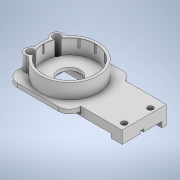
# Autodesk Inventor part: мотор_плеча_1.1
Saved by Autodesk Inventor 2022 (Build 260153000, 153)
## iProperties
Created: 2022-12-03
Part Number: мотор_плеча_1.1
Material: Типовые
Document SubType Name: Modeling
Designer: Папа
Density: 1 g/cm^3
Appearance: По умолчанию
Author: Папа
Autodesk Inventor part; units mm, degrees
ref_plane "YZ Plane" through (0, 0, 0) normal (1, 0, 0) x (0, 1, 0)
ref_plane "XZ Plane" through (0, 0, 0) normal (0, 1, 0) x (-1, 0, 0)
ref_plane "XY Plane" through (0, 0, 0) normal (0, 0, 1) x (1, 0, 0)
sketch "Эскиз1" plane through (0, 0, 0) normal (0, 1, 0) x (-1, 0, 0)
  arc A0 (-2.6622, -14.05) -> (-2.6622, 14.05) centre (0, 0) ccw
  line L0 (-2.6622, 14.05) -> (-34.2422, 14.05)
  line L1 (-34.2422, -14.05) -> (-2.6622, -14.05)
  arc A1 (-34.2422, 6.025) -> (-34.2422, -6.025) centre (-34.2422, 0) ccw
  line L2 (0, 0) -> (-101.5894, 0) construction
  line L3 (-34.2422, 14.05) -> (-34.2422, 6.025)
  line L4 (-34.2422, -6.025) -> (-34.2422, -14.05)
  line L5 (-52.75, 14.55) -> (22.25, 14.55)
  line L6 (22.25, 14.55) -> (22.25, -14.55)
  line L7 (22.25, -14.55) -> (-52.75, -14.55)
  line L8 (-52.75, -14.55) -> (-52.75, 14.55)
  line L9 (-52.75, 14.55) -> (22.25, -14.55) construction
  line L10 (22.25, 14.55) -> (-52.75, -14.55) construction
  line L11 (14.3, 0) -> (22.25, 0)
  line L12 (-34.2422, 6.025) -> (-34.2422, -6.025) construction
  line L13 (22.25, -14.55) -> (-52.75, -14.55)
  line L14 (-52.75, -14.55) -> (-52.75, -17.55)
  line L15 (-52.75, -17.55) -> (22.25, -17.55)
  line L16 (22.25, -17.55) -> (22.25, -14.55)
  point P0 (-15.25, 0)
  dimension "d0" = 28.6
  dimension "d2" = 12.05
  dimension "d4" = 31.58
  dimension "d5" = 14.05
  dimension "d9" = 29.1
  dimension "d10" = 75
  dimension "d12" = 3
  dimension "d25" = 22.25
  constraints: 34 end point, 5 horizontal, 5 point on circle, 4 collinear, 4 midpoint, 4 parallel, 4 perpendicular, 2 centre point, 2 point on line, 1 coincident
  measures "d0" diameter of A0
  measures "d2" diameter of A1
  measures "d4" distance of L1.start L1.end
  measures "d5" distance between parallel lines of L1 L2
  measures "d9" distance between parallel lines of L5 L7
  measures "d10" distance of L6.end L7.end
  measures "d12" distance of L15.end L6.end
  measures "d25" distance from line of L6 point (0, 0)
extrude "Выдавливание2" add sketch "Эскиз1" along normal blind 4
sketch "Эскиз2" plane through (0, 4, 0) normal (0, 1, 0) x (1, 0, 0)
  circle A0 centre (-18.75, -9.5) radius 2.05
  circle A1 centre (-18.75, 9.5) radius 2.05
  circle A2 centre (49.25, -9.5) radius 2.05
  circle A3 centre (49.25, 9.5) radius 2.05
  line L0 (-18.75, -9.5) -> (49.25, -9.5) construction
  line L1 (49.25, -9.5) -> (49.25, 9.5) construction
  line L2 (49.25, 9.5) -> (-18.75, 9.5) construction
  line L3 (-18.75, 9.5) -> (-18.75, -9.5) construction
  line L4 (52.75, -14.55) -> (52.75, 17.55) projected
  line L5 (52.75, -14.55) -> (52.75, 17.55)
  line L6 (-22.25, 17.55) -> (-22.25, -14.55) projected
  line L7 (-22.25, -14.55) -> (52.75, -14.55) projected
  line L8 (34.2422, -14.05) -> (2.6622, -14.05) projected
  line L9 (2.6622, 14.05) -> (34.2422, 14.05) projected
  line L10 (2.6622, -14.05) -> (2.6622, 14.05) construction
  line L11 (2.6622, 0) -> (-18.75, 0)
  point P0 (0, 0)
  dimension "d15" = 4.1
  dimension "d16" = 19
  dimension "d17" = 68
  dimension "d21" = 3.5
  constraints: 14 end point, 4 centre point, 3 equal radius, 2 coincident, 2 midpoint, 2 parallel, 2 perpendicular, 1 horizontal, 1 vertical
  measures "d15" diameter of A0
  measures "d16" distance of L2.end L0.start
  measures "d17" distance of L1.end L2.end
  measures "d21" distance between parallel lines of L6 L3
extrude "Выдавливание3" cut sketch "Эскиз2" against normal blind 4.1
sketch "Эскиз9" plane through (0, 4, 0) normal (0, 1, 0) x (1, 0, 0)
  circle A0 centre (-18.75, -9.5) radius 2.05 projected
  circle A1 centre (-18.75, -9.5) radius 2.05
  circle A2 centre (-18.75, 9.5) radius 2.05 projected
  circle A3 centre (-18.75, 9.5) radius 2.05
  circle A4 centre (49.25, 9.5) radius 2.05 projected
  circle A5 centre (49.25, 9.5) radius 2.05
  circle A6 centre (49.25, -9.5) radius 2.05 projected
  circle A7 centre (49.25, -9.5) radius 2.05
  line L0 (-22.25, -14.55) -> (52.75, -14.55) projected
  line L1 (52.75, -14.55) -> (52.75, 17.55) projected
  line L2 (-22.25, -14.55) -> (52.75, -14.55)
  line L3 (52.75, -14.55) -> (52.75, 17.55)
  line L4 (52.75, 17.55) -> (-22.25, 17.55)
  line L5 (-22.25, 17.55) -> (-22.25, -14.55)
  circle A8 centre (0, 0) radius 8
  line L6 (-18.75, -9.5) -> (-18.75, 9.5) construction
  line L7 (34.2422, -14.05) -> (2.6622, -14.05) projected
  line L8 (2.6622, 14.05) -> (34.2422, 14.05) projected
  line L9 (10.1489, -14.05) -> (10.1489, 14.05)
  dimension "d70" = 16
  dimension "d120" = 18.75
  constraints: 12 end point, 5 centre point, 4 coincident, 2 parallel, 2 perpendicular, 2 point on line, 1 horizontal, 1 vertical
  measures "d70" diameter of A8
  measures "d120" distance from line of A8.centre L6
extrude "Выдавливание11" add sketch "Эскиз9" along normal blind 2.1
sketch "Эскиз10" plane through (0, 0, 0) normal (0, -1, 0) x (1, 0, 0)
  line L0 (52.75, -17.55) -> (-22.25, -17.55) projected
  line L1 (-22.25, -17.55) -> (52.75, -17.55)
  line L2 (52.75, -17.55) -> (52.75, 14.55)
  line L3 (52.75, 14.55) -> (-22.25, 14.55)
  line L4 (-22.25, 14.55) -> (-22.25, -17.55)
  circle A0 centre (-18.75, -9.5) radius 2.05 projected
  circle A1 centre (-18.75, -9.5) radius 2.05
  circle A2 centre (-18.75, 9.5) radius 2.05 projected
  circle A3 centre (-18.75, 9.5) radius 2.05
  circle A4 centre (49.25, 9.5) radius 2.05 projected
  circle A5 centre (49.25, 9.5) radius 2.05
  circle A6 centre (49.25, -9.5) radius 2.05 projected
  circle A7 centre (49.25, -9.5) radius 2.05
  arc A8 (2.6622, 14.05) -> (2.6622, -14.05) centre (0, 0) ccw projected
  circle A9 centre (0, 0) radius 14.3
  line L5 (-22.25, 14.55) -> (52.75, 14.55) projected
  line L6 (-14.275, 14.55) -> (44.775, 14.55)
  line L7 (44.775, 14.55) -> (44.775, -14.3)
  line L8 (44.775, -14.3) -> (-14.275, -14.3)
  line L9 (-14.275, -14.3) -> (-14.275, 14.55)
  point P0 (-14.275, -0.8452)
  point P1 (-14.275, 0.8452)
  dimension "d74" = 59.05
  dimension "d75" = 28.6
  dimension "d76" = 4.475
  constraints: 16 end point, 5 centre point, 5 coincident, 4 parallel, 2 horizontal, 2 perpendicular, 1 point on line, 1 tangent
  measures "d74" distance between parallel lines of L7 L9
  measures "d75" diameter of A9
  measures "d76" distance from line of L9 A1.centre
extrude "Выдавливание12" add sketch "Эскиз10" along normal blind 3 contours L0 L4 L3 L9 A8 L8 L7 L2
sketch "Эскиз11" plane through (0, -3, 0) normal (0, -1, 0) x (1, 0, 0)
  line L0 (52.75, -17.55) -> (-22.25, -17.55) projected
  line L1 (-22.25, -17.55) -> (-22.25, 14.55) projected
  line L2 (52.75, -17.55) -> (-22.25, -17.55)
  line L3 (-22.25, -17.55) -> (-22.25, -14.2815)
  line L4 (-22.25, -14.2815) -> (52.75, -14.2815)
  line L5 (52.75, -14.2815) -> (52.75, -17.55)
  point P0 (0, 0)
  constraints: 8 end point, 2 parallel, 1 horizontal, 1 perpendicular, 1 point on line
extrude "Выдавливание13" add sketch "Эскиз11" along normal blind 4
sketch "Эскиз12" plane through (0, -3, 0) normal (0, -1, 0) x (1, 0, 0)
  circle A0 centre (-18.75, -9.5) radius 2.05 projected
  line L0 (-18.75, -9.5) -> (-18.75, 0) construction
  circle A1 centre (-18.75, 9.5) radius 2.05 projected
  line L1 (-18.75, 0) -> (-18.75, 9.5) construction
  line L2 (-22.25, 14.55) -> (-22.25, -14.2815) projected
  line L3 (-14.9, 1.1) -> (-22.25, 1.1)
  line L4 (-22.25, 1.1) -> (-22.25, -1)
  line L5 (-22.25, -1) -> (-15.5682, -1)
  line L6 (-14.9, 1.1) -> (-22.25, -1) construction
  line L7 (-22.25, 1.1) -> (-15.5682, -1) construction
  line L8 (-14.275, 0.8452) -> (-14.275, 14.55) projected
  line L9 (-15.5682, -1) -> (-14.275, -1)
  line L10 (-14.275, -1) -> (-14.275, 1.1)
  line L11 (-14.275, 1.1) -> (-15.25, 1.1)
  point P0 (0, 0)
  dimension "d82" = 2.1
  constraints: 20 end point, 4 point on line, 3 collinear, 2 horizontal, 2 parallel, 2 perpendicular, 1 vertical
  measures "d82" distance between parallel lines of L11 L9
extrude "Выдавливание14" cut sketch "Эскиз12" against normal blind 2 contours L3 L11 L8 L10 L9 L5 L2
ref_plane "РабПлоскость2" through (15.25, -3, 14.55) normal (-1, 0, 0) x (0, 0, 1)
mirror "Зеркальное отражение2" about plane through (15.25, -3, 14.55) normal (-1, 0, 0) of "Выдавливание14"
sketch "Эскиз13" plane through (0, 6.1, 0) normal (0, 1, 0) x (1, 0, 0)
  circle A0 centre (0, 0) radius 18.9
  circle A1 centre (0, 0) radius 20.9
  dimension "d85" = 37.8
  dimension "d86" = 2
  constraints: 2 centre point, 2 coincident
  measures "d85" diameter of A0
  measures "d86" radial gap between concentric circles of A0 A1
extrude "Выдавливание15" add sketch "Эскиз13" along normal blind 11
sketch "Эскиз15" plane through (0, 6.1, 0) normal (0, 1, 0) x (1, 0, 0)
  circle A0 centre (0, 0) radius 20.9 projected
  circle A1 centre (0, 0) radius 22.9 construction
  line L0 (22.9, -22.9) -> (-22.9, -22.9)
  line L1 (-22.9, -22.9) -> (-22.9, 22.9)
  line L2 (-22.9, 22.9) -> (22.9, 22.9)
  line L3 (22.9, 22.9) -> (22.9, -22.9)
  line L4 (22.9, -22.9) -> (-22.9, 22.9) construction
  line L5 (-22.9, -22.9) -> (22.9, 22.9) construction
  line L6 (-14.275, -14.55) -> (44.775, -14.55) projected
  line L7 (22.9, -14.55) -> (-22.25, -14.55)
  line L8 (-22.25, -14.55) -> (-22.25, 17.55)
  line L9 (-22.25, 17.55) -> (22.9, 17.55)
  line L10 (22.9, 17.55) -> (22.9, -14.55)
  point P0 (-11.3493, 17.55)
  point P1 (11.3493, 17.55)
  point P2 (22.9, 17.55)
  dimension "d91" = 2
  constraints: 20 end point, 4 parallel, 2 horizontal, 2 midpoint, 2 perpendicular, 2 point on line, 2 tangent, 1 centre point, 1 coincident
  measures "d91" radial gap between concentric circles of A1 A0
extrude "Выдавливание18" add sketch "Эскиз15" against normal blind 3 contours L9 A0 | A0 L9 L8 L7 L6 L3 L0 L1 L2 | A0 L7 L6
fillet "Сопряжение5" radius 2 3 edges at (0.325, 3.1, -17.55) (-22.25, 3.1, -1.5) (0.325, 3.1, 14.55)
sketch "Эскиз16" plane through (0, 17.1, 0) normal (0, 1, 0) x (1, 0, 0)
  circle A0 centre (0, 0) radius 18.9 projected
  circle A1 centre (0, 0) radius 18.9 projected
  circle A2 centre (18.9, 0) radius 0.25
  dimension "d99" = 0.5
  constraints: 1 centre point, 1 horizontal alignment, 1 other
  measures "d99" diameter of A2
extrude "Выдавливание19" add sketch "Эскиз16" against normal up to surface (11 mm away) contours A0 A2 | A0 A2 picked at (18.822, -0.0572) picked at (18.975, -0.0641)
fillet "Сопряжение6" radius 0.7 2 edges at (18.8983, 11.6, 0.25) (18.8983, 11.6, -0.25)
pattern_circular "Круговой массив1" count 12 over 360 about axis through (0, 4, 0) along (0, 1, 0) of "Сопряжение6", "Выдавливание19"
sketch "Эскиз17" plane through (0, 6.1, 0) normal (0, 1, 0) x (1, 0, 0)
  arc A0 (-19.4759, -7.5828) -> (-17.6334, -11.2192) centre (-18.75, -9.5) ccw projected
  arc A1 (-17.6334, 11.2192) -> (-19.4759, 7.5828) centre (-18.75, 9.5) ccw projected
  circle A2 centre (-18.75, -9.5) radius 2.8
  arc A3 (-17.6334, -11.2192) -> (-19.4759, -7.5828) centre (-18.75, -9.5) ccw projected
  circle A4 centre (-18.75, 9.5) radius 2.8
  point P0 (0, 0)
  point P1 (-17.611, -11.2545)
  point P2 (-19.4589, -7.6265)
  dimension "d109" = 5.6
  constraints: 2 centre point, 2 coincident, 1 equal radius
  measures "d109" diameter of A2
extrude "Выдавливание20" cut sketch "Эскиз17" along normal blind 4100 and the other way blind 1 contours A3 A0 | A2 | A4
sketch "Эскиз18" plane through (0, 17.1, 0) normal (0, 1, 0) x (1, 0, 0)
  arc A0 (-19.7354, 6.8791) -> (-17.5718, 6.9599) centre (-18.75, 9.5) ccw projected
  circle A1 centre (-18.75, 9.5) radius 2.8
  arc A2 (-19.7354, 6.8791) -> (-19.7354, -6.8791) centre (0, 0) ccw projected
  circle A3 centre (-18.75, -9.5) radius 2.05 projected
  circle A4 centre (-18.75, -9.5) radius 2.8
  arc A5 (-17.2195, -11.8447) -> (-16.005, -10.0523) centre (-18.75, -9.5) ccw projected
  circle A6 centre (-18.75, 9.5) radius 4.15
  circle A7 centre (-18.75, -9.5) radius 4.15
  line L0 (-22.9, 22.9) -> (-22.9, -22.9) projected
  circle A8 centre (0, 0) radius 20.9
  point P0 (-17.2195, 11.8447)
  point P1 (-16.0725, 10.3191)
  point P2 (-16.512, 11.1827)
  point P3 (-18.7831, -6.7002)
  point P4 (-17.8269, -6.8565)
  point P5 (-20.9, 0)
  point P6 (-17.2195, 11.8447)
  point P7 (-16.418, 12.9328)
  point P8 (-20.1388, 5.5893)
  point P9 (-19.7354, 6.8791)
  point P10 (-16.418, -12.9328)
  point P11 (-17.2195, -11.8447)
  point P12 (-20.1388, -5.5893)
  constraints: 5 coincident, 5 point on circle, 4 centre point, 2 tangent, 3 other
extrude "Выдавливание21" add sketch "Эскиз18" against normal up to surface (11 mm away) contours A2 A6 A8 A1 | A2 A4 A8 A7 picked at (-22.2151, -8.2781)
fillet "Сопряжение8" radius 2 4 edges at (-16.418, 11.6, -12.9328) (-20.1388, 11.6, 5.5893) (-16.418, 11.6, 12.9328) (-20.1388, 11.6, -5.5893)
fillet "Сопряжение9" radius 8 4 edges at (-22.9, 4.6, -22.9) (22.9, 4.6, -22.9) (22.9, 4.6, 22.9) (-22.9, 4.6, 22.9)
ref_plane "РабПлоскость4" through (-14.275, -3, 0.05) normal (0, 0, -1) x (-1, 0, 0)
sketch "Эскиз23" plane through (0, 6.1, 0) normal (0, 1, 0) x (1, 0, 0)
  circle A0 centre (0, 0) radius 18.9
  circle A1 centre (-18.75, -9.5) radius 2.05 projected
  circle A2 centre (-18.75, -9.5) radius 2.8
  arc A3 (-16.005, -10.0523) -> (-17.5718, -6.9599) centre (-18.75, -9.5) ccw projected
  arc A4 (-17.5718, 6.9599) -> (-18.8887, 0.6544) centre (0, 0) ccw projected
  circle A5 centre (-18.75, 9.5) radius 2.8
  circle A6 centre (0, 0) radius 8
  point P0 (-18.8887, -0.6544)
  point P1 (-16.005, 10.0523)
  point P2 (-16.005, -10.0523)
  dimension "d133" = 16
  constraints: 4 coincident, 2 centre point, 1 point on circle, 6 other
  measures "d133" diameter of A6
extrude "Выдавливание26" add sketch "Эскиз23" along normal blind 0.2 contours A5 A0 A2
fillet "Сопряжение10" radius 0.2 42 edges at (-18.8478, 17.1, 0.3932) (-18.65, 17.1, 0) (-18.8478, 17.1, -0.3932) (-18.5009, 17.1, -3.8637) (-18.5009, 17.1, 3.8637) (-9.7644, 17.1, 16.126) (-9.325, 17.1, 16.1514) (-9.0833, 17.1, 16.5193) (-4.8917, 17.1, 18.256) (-0.3932, 17.1, 18.8478) (0, 17.1, 18.65) (0.3932, 17.1, 18.8478) (4.8917, 17.1, 18.256) (9.0833, 17.1, 16.5193) (9.325, 17.1, 16.1514) (9.7644, 17.1, 16.126) (13.3643, 17.1, 13.3643) (16.126, 17.1, 9.7644) (16.1514, 17.1, 9.325) (16.5193, 17.1, 9.0833) (18.256, 17.1, 4.8917) (18.8478, 17.1, 0.3932) (18.65, 17.1, 0) (18.8478, 17.1, -0.3932) (18.256, 17.1, -4.8917) (16.5193, 17.1, -9.0833) (16.1514, 17.1, -9.325) (16.126, 17.1, -9.7644) (13.3643, 17.1, -13.3643) (9.7644, 17.1, -16.126) (9.325, 17.1, -16.1514) (9.0833, 17.1, -16.5193) (4.8917, 17.1, -18.256) (0.3932, 17.1, -18.8478) (0, 17.1, -18.65) (-0.3932, 17.1, -18.8478) (-4.8917, 17.1, -18.256) (-9.0833, 17.1, -16.5193) (-9.325, 17.1, -16.1514) (-9.7644, 17.1, -16.126) (-13.3471, 17.1, -13.3815) (-13.3471, 17.1, 13.3815)
sketch "Эскиз24" plane through (0, 6.3, 0) normal (0, 1, 0) x (1, 0, 0)
  circle A0 centre (0, 0) radius 18.9
  constraints: 1 centre point, 1 coincident
extrude "Выдавливание27" cut sketch "Эскиз24" along normal blind 4.8
